Autodesk Inventor part; units mm, degrees
(part 4 of 4)
extrude "Extrusão3" cut sketch "Esboço3" against normal blind 0.1 bodies 2
